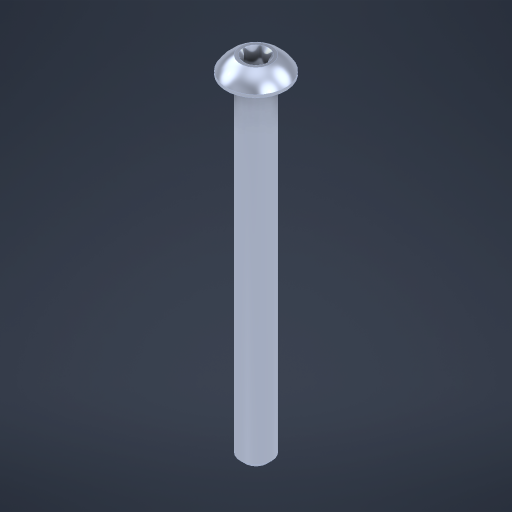
# Autodesk Inventor part: SScrew Shoulder Smooth 1.750 x .04
Saved by Autodesk Inventor 2024 (Build 280153000, 153)
## iProperties
Created: 2020-07-03
Part Number: SScrew Shoulder Smooth 1.750 x .04
Material: VEX Steel
Document SubType Name: Modeling
Designer: yuany
Density: 1 g/cm^3
Appearance: VEX Steel
Author: yuany
Autodesk Inventor part; units mm, degrees
ref_plane "YZ Plane" through (0, 0, 0) normal (1, 0, 0) x (0, 1, 0)
ref_plane "XZ Plane" through (0, 0, 0) normal (0, 1, 0) x (-1, 0, 0)
ref_plane "XY Plane" through (0, 0, 0) normal (0, 0, 1) x (1, 0, 0)
sketch "Sketch1" plane through (0, 0, 0) normal (0, 1, 0) x (-1, 0, 0)
  circle A0 centre (0, 0) radius 2.0828
  dimension "d4" = 4.1656
  constraints: 1 centre point, 1 coincident
  measures "d4" diameter of A0
extrude "Body" add sketch "Sketch1" along normal blind 44.45
sketch "Sketch2" plane through (0, 0, 0) normal (1, 0, 0) x (0, 1, 0)
  line L0 (44.45, -2.0828) -> (44.45, 2.0828) projected
  line L1 (44.45, 0) -> (44.45, -3.9624)
  line L2 (44.45, -3.9624) -> (44.831, -3.9624)
  arc A0 (44.831, -3.9624) -> (46.6598, -2.0828) centre (42.6388, 0) ccw
  line L3 (46.6598, -2.0828) -> (46.6598, -1.6764)
  line L4 (46.6598, -1.6764) -> (45.1635, -1.6764)
  line L5 (45.1635, -1.6764) -> (44.5516, 0)
  line L6 (44.5516, 0) -> (44.45, 0)
  point P0 (0, 0)
  dimension "d5" = 3.9624
  dimension "d6" = 0.381
  dimension "d13" = 0.1016
  dimension "d14" = 2.0828
  dimension "d15" = 2.2098
  dimension "d16" = 0
  dimension "d17" = 1.6764
  dimension "d57" = 20.053
  constraints: 12 end point, 2 horizontal, 2 point on circle, 1 centre point, 1 midpoint, 1 perpendicular, 1 point on line, 1 vertical
  measures "d5" distance of L1.start L1.end
  measures "d6" distance of L1.end L2.end
  measures "d13" distance of L5.end L1.start
  measures "d14" distance from line of L3.start L6
  measures "d15" distance between parallel lines of L1 L3
  measures "d16" distance from line of L6 A0.centre
  measures "d17" distance from line of L3.end L6
  measures "d57" angle of L1 L5
revolve "Head" add sketch "Sketch2" angle 360 about axis through (0, 44.5516, 0) along (0, -1, 0)
sketch "Sketch3" plane through (0, 46.6598, 0) normal (0, 1, 0) x (1, 0, 0)
  circle A0 centre (0, 0) radius 1.6764 projected
  line L0 (0.7302, -1.2648) -> (-0.7303, -1.2648) construction
  line L1 (-0.7303, -1.2648) -> (-1.4605, 0) construction
  line L2 (-1.4605, 0) -> (-0.7303, 1.2648) construction
  line L3 (-0.7303, 1.2648) -> (0.7302, 1.2648) construction
  line L4 (0.7302, 1.2648) -> (1.4605, 0) construction
  line L5 (1.4605, 0) -> (0.7302, -1.2648) construction
  circle A1 centre (-0.7303, -1.2648) radius 0.2159
  circle A2 centre (-1.4605, 0) radius 0.2159
  circle A3 centre (-0.7303, 1.2648) radius 0.2159
  circle A4 centre (0.7302, 1.2648) radius 0.2159
  circle A5 centre (1.4605, 0) radius 0.2159
  circle A6 centre (0.7302, -1.2648) radius 0.2159
  circle A7 centre (0, -2.0701) radius 0.8712
  circle A8 centre (0, 2.0701) radius 0.8712
  circle A9 centre (1.7928, -1.0351) radius 0.8712
  circle A10 centre (-1.7928, 1.035) radius 0.8712
  circle A11 centre (1.7928, 1.035) radius 0.8712
  circle A12 centre (-1.7928, -1.0351) radius 0.8712
  circle A13 centre (0, 0) radius 1.8188
  point P0 (0, 0)
  point P1 (0, 0)
  point P2 (0.9413, 1.2192)
  point P3 (1.5265, 0.2056)
  point P4 (1.5265, -0.2056)
  point P5 (0.9413, -1.2192)
  point P6 (0.5852, -1.4248)
  point P7 (-0.5852, -1.4248)
  point P8 (-0.9413, -1.2192)
  point P9 (-1.5265, -0.2056)
  point P10 (-1.5265, 0.2056)
  point P11 (-0.9413, 1.2192)
  point P12 (-0.5852, 1.4248)
  point P13 (0.5852, 1.4248)
  dimension "d58" = 2.921
  dimension "d59" = 4.1402
  dimension "d62" = 120
  constraints: 13 centre point, 12 end point, 10 tangent, 9 coincident, 1 equal radius, 1 horizontal, 22 other
  measures "d58" distance of L0.end L3.end
  measures "d59" distance of A7.centre A8.centre
extrude "Hex" add sketch "Sketch3" against normal blind 1.778 contours A5 A11 A0 | A0 A11 A13 A9 | A0 A9 A5 | A11 A0 | A0 A11 A13 | A9 A13 A0 | A0 A9 | A11 A4 A0 | A0 A8 A13 A11 | A9 A13 A7 A0 | A0 A6 A9 | A4 A8 A0 | A0 A7 A6 | A8 A0 | A7 A0 | A0 A8 A13 | A7 A13 A0 | A3 A0 A8 | A7 A0 A1 | A0 A10 A13 A8 | A7 A13 A12 A0 | A3 A10 A0 | A0 A12 A1 | A10 A0 A13 | A13 A12 A0 | A10 A0 | A0 A12 | A10 A0 A12 A13 | A10 A2 A0 | A0 A2 A12
sketch "Sketch4" plane through (0, 0, 0) normal (0, 0, 1) x (1, 0, 0)
  line L0 (-0.7364, 45.7198) -> (-1.6764, 46.6598)
  line L1 (0, 46.6598) -> (-0.7364, 45.7198)
  line L2 (0, -10.602) -> (0, 63.6118) projected
  line L3 (-1.5265, 46.6598) -> (-1.5265, 45.1138) projected
  line L4 (-1.5265, 46.6598) -> (-1.5265, 46.6598) projected
  line L5 (-1.5265, 46.6598) -> (-1.5265, 45.1138) projected
  line L6 (-1.6764, 46.6598) -> (-1.5265, 46.6598) projected
  line L7 (-1.6764, 46.6598) -> (0, 46.6598)
  point P0 (0, 0)
  dimension "d29" = 1.6764
  constraints: 6 end point, 1 horizontal, 2 other
  measures "d29" distance of L0.end L1.start
revolve "Head Chamfer" cut sketch "Sketch4" angle 360 about axis through (0, -10, 0) along (0, 1, 0)
feature "Thread" [suppressed]
sketch "Sketch6" plane through (0, 0, 0) normal (0, 0, 1) x (1, 0, 0)
  line L0 (0, 0) -> (-1.4859, 0)
  line L1 (2.0828, 0) -> (-2.0828, 0) projected
  line L2 (-1.4859, 0) -> (-2.4948, 1.0089)
  line L3 (-2.4948, 1.0089) -> (-2.9651, -1.2188)
  line L4 (-2.9651, -1.2188) -> (-1.4859, -1.2188)
  line L5 (-2.0828, 0) -> (-2.0828, 44.45) projected
  line L6 (-1.4859, -1.2188) -> (-1.4859, 0)
  line L7 (0, -11.6226) -> (0, 61.2038) projected
  point P0 (-2.0828, 0.5969)
  dimension "d49" = 1.4859
  dimension "d50" = 135
  constraints: 10 end point, 1 perpendicular, 1 point on line, 1 vertical
  measures "d49" distance from line of L0.start L6
  measures "d50" angle of L2 L6
revolve "Tapered End" cut sketch "Sketch6" angle 360 about axis through (0, -10, 0) along (0, 1, 0)
sketch "Sketch8" plane through (0, 0, 0) normal (0, 0, 1) x (1, 0, 0)
  line L0 (-3.9624, 44.45) -> (3.9624, 44.45) projected
  line L1 (0, 44.45) -> (2.286, 44.45)
  line L2 (2.286, 44.45) -> (2.286, 43.434)
  line L3 (2.286, 43.434) -> (0, 43.434)
  line L4 (0, 43.434) -> (0, 44.45)
  point P0 (0, 0)
  dimension "d69" = 2.286
  dimension "d70" = 1.016
  constraints: 8 end point, 2 parallel, 1 horizontal, 1 midpoint, 1 perpendicular
  measures "d69" distance of L2.end L3.end
  measures "d70" distance of L1.end L2.end
revolve "Shoulder" add sketch "Sketch8" angle 360 about axis through (0, 43.434, 0) along (0, 1, 0)
sketch "Sketch5" plane through (0, 0, 0) normal (1, 0, 0) x (0, 1, 0)
  line L0 (0, -2.0828) -> (44.45, -2.0828) projected
  line L1 (44.45, 3.9624) -> (44.45, -3.9624) projected
  line L2 (44.45, -2.0828) -> (44.45, 2.0828) projected
  line L3 (0.0745, -2.0828) -> (-0.2261, -2.6035)
  line L4 (-0.2261, -2.6035) -> (-0.3253, -2.6035)
  line L5 (-0.3253, -2.6035) -> (-0.626, -2.0828)
  line L6 (0.0686, -2.6035) -> (-0.7252, -2.6035) construction
  line L7 (-0.626, -2.0828) -> (0.0745, -2.0828)
  line L8 (0, -2.0828) -> (44.45, -2.0828) projected
  point P0 (0, 0)
  dimension "d31" = 30
  dimension "d32" = 60
  dimension "a" = 0.0992
  dimension "d46" = 0.7937
  dimension "d54" = 0.0686
  dimension "d55" = 0.5207
  dimension "d56" = 0.0992
  constraints: 10 end point, 2 collinear, 2 point on line, 1 horizontal, 1 perpendicular
  measures "d31" angle of L1 L3
  measures "d32" angle of L3 L5
  measures "a" distance of L3.end L4.end
  measures "d46" distance of L6.start L6.end
  measures "d54" horizontal distance of L6.start L8.start
  measures "d55" distance between parallel lines of L4 L7
  measures "d56" horizontal distance of L5.end L6.end
equation "\"d56\" = a"
equation "\"ShoulderLength\" = 1.016"
body "Solid1"
